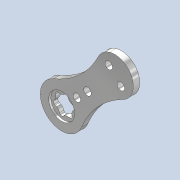
# Autodesk Inventor part: 原動節
Saved by Autodesk Inventor 2020.4 (Build 244396000, 396)
## iProperties
Created: 2021-04-23
Part Number: 原動節
Material: アルミニウム 2014-T4
Document SubType Name: Modeling
Designer: happy
Density: 2.8 g/cm^3
Appearance: サテン
Mass: 5.64562 g
Surface Area: 20.029 cm^2
Volume: 2.01629 cm^3
Author: happy
Autodesk Inventor part; units mm, degrees
ref_plane "YZ Plane" through (0, 0, 0) normal (1, 0, 0) x (0, 1, 0)
ref_plane "XZ Plane" through (0, 0, 0) normal (0, 1, 0) x (-1, 0, 0)
ref_plane "XY Plane" through (0, 0, 0) normal (0, 0, 1) x (1, 0, 0)
sketch "スケッチ1" plane through (0, 0, 0) normal (0, 0, 1) x (1, 0, 0)
  line L0 (0, 0) -> (24.7487, 24.7487) construction
  line L1 (0, 0) -> (8.6903, 0) construction
  circle A0 centre (7.0711, 7.0711) radius 1.75
  circle A1 centre (12.0208, 12.0208) radius 1.75
  circle A2 centre (24.7487, 24.7487) radius 4.6188 construction
  circle A3 centre (24.7487, 24.7487) radius 8.6188
  line L2 (21.4828, 21.4828) -> (28.0147, 28.0147) construction
  circle A4 centre (29.2102, 23.5533) radius 4 construction
  circle A5 centre (21.4828, 21.4828) radius 4 construction
  circle A6 centre (23.5533, 29.2102) radius 4 construction
  circle A7 centre (29.2102, 23.5533) radius 1.5
  circle A8 centre (21.4828, 21.4828) radius 1.5
  circle A9 centre (23.5533, 29.2102) radius 1.5
  circle A10 centre (24.7487, 24.7487) radius 0.8755 construction
  circle A11 centre (0, 0) radius 5 construction
  arc A12 (5.7301, 8.1955) -> (7.0711, 7.0711) centre (0, 0) ccw
  arc A13 (-3.7643, 9.2644) -> (17.0249, 28.5731) centre (-18.8216, 46.3222) ccw
  arc A14 (28.5731, 17.0249) -> (9.2644, -3.7643) centre (46.3222, -18.8216) ccw
  line L3 (-4.8296, -1.2941) -> (-3.5355, 3.5355) construction
  line L4 (-3.5355, 3.5355) -> (1.2941, 4.8296) construction
  line L5 (1.2941, 4.8296) -> (4.8296, 1.2941) construction
  line L6 (4.8296, 1.2941) -> (3.5355, -3.5355) construction
  line L7 (3.5355, -3.5355) -> (-1.2941, -4.8296) construction
  line L8 (-1.2941, -4.8296) -> (-4.8296, -1.2941) construction
  arc A15 (-2.5213, 3.8073) -> (-3.8073, 2.5213) centre (-2.7931, 2.7931) ccw
  arc A16 (-4.5579, -0.2799) -> (-4.0872, -2.0366) centre (-3.8154, -1.0223) ccw
  arc A17 (-2.0366, -4.0872) -> (-0.2799, -4.5579) centre (-1.0223, -3.8154) ccw
  arc A18 (2.5213, -3.8073) -> (3.8073, -2.5213) centre (2.7931, -2.7931) ccw
  arc A19 (4.5579, 0.2799) -> (4.0872, 2.0366) centre (3.8154, 1.0223) ccw
  arc A20 (2.0366, 4.0872) -> (0.2799, 4.5579) centre (1.0223, 3.8154) ccw
  arc A21 (-2.5213, 3.8073) -> (0.2799, 4.5579) centre (-1.7707, 6.6085) ccw
  arc A22 (-4.5579, -0.2799) -> (-3.8073, 2.5213) centre (-6.6085, 1.7707) ccw
  arc A23 (-2.0366, -4.0872) -> (-4.0872, -2.0366) centre (-4.8377, -4.8377) ccw
  arc A24 (2.5213, -3.8073) -> (-0.2799, -4.5579) centre (1.7707, -6.6085) ccw
  arc A25 (4.5579, 0.2799) -> (3.8073, -2.5213) centre (6.6085, -1.7707) ccw
  arc A26 (2.0366, 4.0872) -> (4.0872, 2.0366) centre (4.8377, 4.8377) ccw
  circle A27 centre (0, 0) radius 6.05
  circle A28 centre (24.7487, 24.7487) radius 4 construction
  circle A29 centre (24.7487, 24.7487) radius 8
  line L9 (21.0131, 23.3188) -> (28.4844, 26.1787) construction
  circle A30 centre (21.9203, 27.5772) radius 4 construction
  circle A31 centre (27.5772, 21.9203) radius 4 construction
  circle A32 centre (21.9203, 27.5772) radius 3
  circle A33 centre (27.5772, 21.9203) radius 3
  line L10 (21.9203, 27.5772) -> (27.5772, 21.9203) construction
  circle A34 centre (21.9203, 27.5772) radius 1.75
  circle A35 centre (27.5772, 21.9203) radius 1.75
  point P0 (220.0202, -53)
  point P1 (-4.8296, -1.2941)
  point P2 (-1.2941, -4.8296)
  point P3 (3.5355, -3.5355)
  point P4 (4.8296, 1.2941)
  point P5 (4.0872, 2.0366)
  point P6 (4.5579, 0.2799)
  point P7 (3.8073, -2.5213)
  point P8 (2.5213, -3.8073)
  point P9 (-0.2799, -4.5579)
  point P10 (-2.0366, -4.0872)
  point P11 (-4.0872, -2.0366)
  point P12 (-4.5579, -0.2799)
  dimension "d2" = 3.5
  dimension "d15" = 10
  dimension "d0" = 35
  dimension "d1" = 45
  dimension "d3" = 3.5
  dimension "d4" = 10
  dimension "d5" = 7
  dimension "d10" = 17.2376
  dimension "d11" = 8
  dimension "d13" = 3
  dimension "d16" = 20
  dimension "d17" = 40
  dimension "d22" = 360
  dimension "d26" = 360
  dimension "d28" = 1.05
  dimension "d29" = 12.1
  dimension "d32" = 16
  dimension "d33" = 8
  dimension "d34" = 6
  dimension "d35" = 6
  dimension "d36" = 3.5
  dimension "d37" = 3.5
  constraints: 50 point on circle, 34 centre point, 22 end point, 15 coincident, 13 tangent, 6 point on line, 5 equal radius, 5 midpoint, 1 concentric, 1 horizontal, 1 perpendicular, 76 other
  measures "d0" distance of L0.start L0.end
  measures "d1" angle of L1 L0
  measures "d3" diameter of A1
  measures "d4" distance of L0.start point (7.071, 7.071)
  measures "d5" distance of A1.centre point (7.071, 7.071)
  measures "d10" diameter of A3
  measures "d11" diameter of A5
  measures "d13" diameter of A8
  measures "d16" diameter of A12
  measures "d17" radius of A13
  measures "d28" radius of A15
  measures "d29" diameter of A27
  measures "d32" diameter of A29
  measures "d33" diameter of A30
  measures "d34" diameter of A32
  measures "d35" diameter of A33
  measures "d36" diameter of A34
  measures "d37" diameter of A35
extrude "押し出し1" add sketch "スケッチ1" along normal blind 3 contours A0 A12 A13 A3 A14 | A0 A12 | A3 | A7 A33 | A33 A7 A35 | A7 A35 A33 | A8 | A9 A32 | A32 A9 A34 | A9 A34 A32 | A27 | A29
sketch "スケッチ2" plane through (0, 0, 3) normal (0, 0, 1) x (1, 0, 0)
  circle A0 centre (0, 0) radius 6.05 projected
extrude "押し出し2" cut sketch "スケッチ2" against normal blind 1
equation "\"d37\" = d36"
